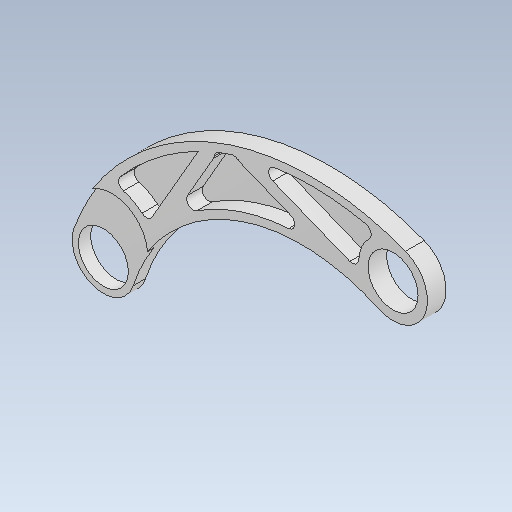
# Autodesk Inventor part: 揺動節六角ver2
Saved by Autodesk Inventor 2020.2 (Build 242310000, 310)
## iProperties
Created: 2019-11-01
Part Number: 揺動節六角ver2
Material: アルミニウム 2014-T4
Document SubType Name: Modeling
Designer: aoyam
Density: 2.8 g/cm^3
Appearance: サテン
Mass: 3.17251 g
Surface Area: 20.2095 cm^2
Volume: 1.13304 cm^3
Author: aoyam
Autodesk Inventor part; units mm, degrees
ref_plane "YZ Plane" through (0, 0, 0) normal (1, 0, 0) x (0, 1, 0)
ref_plane "XZ Plane" through (0, 0, 0) normal (0, 1, 0) x (-1, 0, 0)
ref_plane "XY Plane" through (0, 0, 0) normal (0, 0, 1) x (1, 0, 0)
sketch "スケッチ1" plane through (0, 0, 0) normal (0, 0, 1) x (1, 0, 0)
  line L0 (76.8079, 32.4602) -> (29.2316, 11.4721)
  circle A0 centre (29.2316, 11.4721) radius 4.025
  circle A1 centre (29.2316, 11.4721) radius 5.025
  circle A2 centre (76.8079, 32.4602) radius 4.025
  circle A3 centre (76.8079, 32.4602) radius 5.525
  arc A4 (78.8037, 37.6121) -> (24.523, 13.2269) centre (63.7003, -1.3742) ccw
  arc A5 (74.4764, 27.4512) -> (34.0063, 9.9057) centre (62.0306, 0.7119) ccw
  line L1 (29.2316, 11.4721) -> (80.8221, 4.9588)
  dimension "d0" = 52
  dimension "d1" = 8.05
  dimension "d2" = 1
  dimension "d3" = 8.05
  dimension "d4" = 1.5
  dimension "d7" = 52
  dimension "d8" = 329
  dimension "d9" = 41.8097
  dimension "d10" = 29.4939
  constraints: 8 point on circle, 6 centre point, 4 end point, 4 tangent, 2 coincident
  measures "d0" distance of L0.start L0.end
  measures "d1" diameter of A0
  measures "d2" radial gap between concentric circles of A0 A1
  measures "d3" diameter of A2
  measures "d4" radial gap between concentric circles of A2 A3
  measures "d7" distance of L1.start L1.end
  measures "d9" radius of A4
  measures "d10" radius of A5
extrude "押し出し1" add sketch "スケッチ1" along normal blind 3 contours A3 A5 L0 | L0 A5 A1 A4 A3 | A3 | A5 L1 A1 L0 | A1 L0 A0 L1 | A1 L1 A0 L0 | A5 A1 L1
sketch "スケッチ2" plane through (0, 0, 3) normal (0, 0, 1) x (1, 0, 0)
  arc A0 (78.8037, 37.6121) -> (24.523, 13.2269) centre (63.7003, -1.3742) ccw projected
  arc A1 (24.523, 13.2269) -> (34.0063, 9.9057) centre (29.2316, 11.4721) ccw projected
  arc A2 (74.4764, 27.4512) -> (34.0063, 9.9057) centre (62.0306, 0.7119) ccw projected
  arc A3 (74.4764, 27.4512) -> (78.8037, 37.6121) centre (76.8079, 32.4602) ccw projected
  circle A4 centre (76.8079, 32.4602) radius 4.025 projected
  circle A5 centre (29.2316, 11.4721) radius 4.025 projected
  arc A6 (37.33, 16.8293) -> (28.4907, 21.1721) centre (31.5962, 16.3258) ccw
  arc A7 (78.3522, 36.4465) -> (25.6943, 12.7904) centre (63.7003, -1.3742) ccw
  arc A8 (75.0039, 28.5845) -> (78.3522, 36.4465) centre (76.8079, 32.4602) ccw
  arc A9 (75.0039, 28.5845) -> (32.8185, 10.2953) centre (62.0306, 0.7119) ccw
  arc A10 (25.6943, 12.7904) -> (32.8185, 10.2953) centre (29.2316, 11.4721) ccw
  arc A11 (38.8243, 16.9605) -> (27.6814, 22.4351) centre (31.5962, 16.3258) ccw
  circle A12 centre (76.8079, 32.4602) radius 5.525
  line L0 (37.9515, 19.8269) -> (47.0793, 35.6235) construction
  line L1 (38.8174, 19.3266) -> (47.9452, 35.1232)
  line L2 (46.2135, 36.1238) -> (37.0857, 20.3272)
  arc A13 (37.0857, 20.3272) -> (38.8174, 19.3266) centre (37.9515, 19.8269) ccw
  arc A14 (47.9452, 35.1232) -> (46.2135, 36.1238) centre (47.0793, 35.6235) ccw
  line L3 (52.5563, 37.6245) -> (71.9612, 29.8078) construction
  line L4 (52.1826, 36.6969) -> (71.5876, 28.8802)
  line L5 (72.3348, 30.7354) -> (52.9299, 38.5521)
  arc A15 (52.9299, 38.5521) -> (52.1826, 36.6969) centre (52.5563, 37.6245) ccw
  arc A16 (71.5876, 28.8802) -> (72.3348, 30.7354) centre (71.9612, 29.8078) ccw
  point P0 (0, 0)
  point P1 (74.8442, 37.6245)
  point P2 (31.7261, 23.5806)
  point P3 (42.5154, 27.7252)
  point P4 (62.2587, 33.7161)
  point P5 (37.3374, 20.7628)
  point P6 (45.4867, 34.866)
  point P7 (54.1741, 38.0509)
  point P8 (71.4556, 31.0895)
  point P9 (51.5982, 37.3379)
  point P10 (47.9965, 36.022)
  point P11 (41.0421, 23.1767)
  point P12 (65.7561, 31.2292)
  dimension "d16" = 1.5
  dimension "d17" = 1.5
  dimension "d25" = 1.25
  dimension "d26" = 2
  dimension "d27" = 2
  constraints: 27 point on circle, 16 end point, 10 centre point, 8 tangent, 2 midpoint, 2 parallel, 7 other
  measures "d16" radial gap between concentric circles of A11 A6
  measures "d25" radial gap between concentric circles of A0 A7
  measures "d26" diameter of A14
  measures "d27" diameter of A16
extrude "押し出し2" cut sketch "スケッチ2" against normal blind 1 contours A6 A7 A5 A9 A2 A1 A0 | A6 A9 A5 A7
extrude "押し出し3" cut sketch "スケッチ2" against normal blind 2.5 contours A7 L2 A11 | A12 L5 A7 | A7 A15 L4 A9 L1 A14
fillet "フィレット1" radius 1.05 2 edges at (31.7261, 23.5806, 1.75) (74.8442, 37.6245, 1.75)
fillet "フィレット2" radius 1.05 7 edges at (37.3374, 20.7628, 1.75) (41.0421, 23.1767, 1.75) (47.9965, 36.022, 1.75) (51.5982, 37.3379, 1.75) (65.7561, 31.2292, 1.75) (71.4556, 31.0895, 1.75) (54.1741, 38.0509, 1.75)
